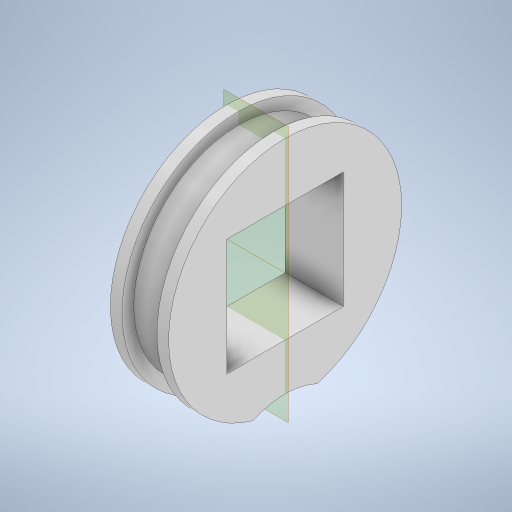
# Autodesk Inventor part: antenna_rad
Saved by Autodesk Inventor 2024 (Build 280153000, 153)
## iProperties
Created: 2025-12-27
Part Number: antenna_rad
Material: PET Plastic
Document SubType Name: Modeling
Designer: schar
Density: 1.541 g/cm^3
Appearance: Polycarbonate - Clear
Author: schar
Autodesk Inventor part; units mm, degrees
ref_plane "YZ Plane" through (0, 0, 0) normal (1, 0, 0) x (0, 1, 0)
ref_plane "XZ Plane" through (0, 0, 0) normal (0, 1, 0) x (-1, 0, 0)
ref_plane "XY Plane" through (0, 0, 0) normal (0, 0, 1) x (1, 0, 0)
sketch "Sketch1" plane through (0, 0, 0) normal (1, 0, 0) x (0, 1, 0)
  line L0 (10, 10) -> (-10, 10)
  line L1 (-10, 10) -> (-10, -10)
  line L2 (-10, -10) -> (10, -10)
  line L3 (10, -10) -> (10, 10)
  line L4 (10, 10) -> (-10, -10) construction
  line L5 (-10, 10) -> (10, -10) construction
  circle A0 centre (0, 0) radius 14.1421
  circle A1 centre (0, 0) radius 20
  dimension "d0" = 20
  dimension "d1" = 20
  dimension "d2" = 40
  constraints: 12 end point, 2 coincident, 2 midpoint, 2 parallel, 1 centre point, 1 horizontal, 1 perpendicular, 3 other
  measures "d0" distance of L2.end L1.end
  measures "d1" distance of L1.end L0.end
  measures "d2" diameter of A1
extrude "Extrusion1" add sketch "Sketch1" along normal blind 10 contours A0 L3 | L0 A0 | L1 A0 | A0 L2 | A1
ref_plane "Work Plane1" through (0, -10, 0) normal (0, 0, -1) x (-1, 0, 0)
sketch "Sketch2" plane through (0, -10, 0) normal (0, 0, -1) x (-1, 0, 0)
  line L0 (0, 30) -> (-10, 30) projected
  line L1 (0, 30) -> (-5, 30)
  line L2 (-5, 30) -> (-2, 30)
  line L3 (-5, 30) -> (-8, 30)
  line L4 (-8, 30) -> (-8, 28)
  line L5 (-8, 28) -> (-3, 28)
  line L6 (-8, 28) -> (-2, 28)
  line L7 (-2, 28) -> (-2, 30)
  line L8 (-2, 30) -> (-8, 30)
  line L9 (-8, 30) -> (-8, 28)
  line L10 (2, 10) -> (-12, 10) projected
  point P0 (0, 10)
  point P1 (-2.5, 28)
  dimension "d5" = 3
  dimension "d6" = 3
  dimension "d7" = 2
  constraints: 18 end point, 3 perpendicular, 3 point on line, 2 parallel, 1 horizontal, 1 midpoint
  measures "d5" distance of L1.end L2.end
  measures "d6" distance of L1.end L3.end
  measures "d7" distance of L3.end L4.end
revolve "Revolution1" cut sketch "Sketch2" angle 360 about axis through (-10, 0, 0) along (1, 0, 0)
sketch "Sketch3" plane through (2, 0, 0) normal (1, 0, 0) x (0, 0, -1)
  circle A0 centre (0, 0) radius 18 projected
  line L0 (0, -18) -> (0, -31)
  circle A1 centre (0, -31) radius 13
  dimension "d9" = 13
  constraints: 2 end point, 2 vertical alignment, 1 coincident, 1 vertical, 3 other
  measures "d9" distance of L0.start L0.end
extrude "Extrusion2" cut sketch "Sketch3" along normal blind 10 contours A1
body "Solid1"
